Autodesk Fusion 360 part; units mm, degrees
(part 8 of 8)
  line L2633 (-418.8503, 9.35) -> (-418.8503, 6.35)
  line L2634 (-418.8503, 6.35) -> (-415.8503, 6.35)
  line L2635 (-415.8503, 6.35) -> (-415.8503, 9.35)
  line L2636 (-415.8503, 9.35) -> (-412.8503, 9.35)
  line L2637 (-412.8503, 9.35) -> (-412.8503, 6.35)
  line L2638 (-412.8503, 6.35) -> (-409.8503, 6.35)
  line L2639 (-409.8503, 6.35) -> (-409.8503, 9.35)
  line L2640 (-409.8503, 9.35) -> (-406.8503, 9.35)
  line L2641 (-406.8503, 9.35) -> (-406.8503, 6.35)
  line L2642 (-406.8503, 6.35) -> (-403.8503, 6.35)
  line L2643 (-403.8503, 6.35) -> (-403.8503, 9.35)
  line L2644 (-403.8503, 9.35) -> (-400.8503, 9.35)
  line L2645 (-400.8503, 9.35) -> (-400.8503, 6.35)
  line L2646 (-400.8503, 6.35) -> (-397.8503, 6.35)
  line L2647 (-397.8503, 6.35) -> (-397.8503, 9.35)
  line L2648 (-397.8503, 9.35) -> (-394.8503, 9.35)
  line L2649 (-394.8503, 9.35) -> (-394.8503, 6.35)
  line L2650 (-394.8503, 6.35) -> (-391.8503, 6.35)
  line L2651 (-391.8503, 6.35) -> (-391.8503, 9.35)
  line L2652 (-391.8503, 9.35) -> (-388.8503, 9.35)
  line L2653 (-388.8503, 9.35) -> (-388.8503, 6.35)
  line L2654 (-388.8503, 6.35) -> (-385.8503, 6.35)
  line L2655 (-385.8503, 6.35) -> (-385.8503, 9.35)
  line L2656 (-385.8503, 9.35) -> (-382.8503, 9.35)
  line L2657 (-382.8503, 9.35) -> (-382.8503, 6.35)
  line L2658 (-382.8503, 6.35) -> (-379.8503, 6.35)
  line L2659 (-379.8503, 6.35) -> (-379.8503, 9.35)
  line L2660 (-379.8503, 9.35) -> (-376.8503, 9.35)
  line L2661 (-376.8503, 9.35) -> (-376.8503, 6.35)
  line L2662 (-376.8503, 6.35) -> (-373.8503, 6.35)
  line L2663 (-373.8503, 6.35) -> (-373.8503, 9.35)
  line L2664 (-373.8503, 9.35) -> (-370.8503, 9.35)
  line L2665 (-370.8503, 9.35) -> (-370.8503, 6.35)
  line L2666 (-370.8503, 6.35) -> (-367.8503, 6.35)
  line L2667 (-367.8503, 6.35) -> (-367.8503, 9.35)
  line L2668 (-367.8503, 9.35) -> (-364.8503, 9.35)
  line L2669 (-364.8503, 9.35) -> (-364.8503, 6.35)
  line L2670 (-364.8503, 6.35) -> (-361.8503, 6.35)
  line L2671 (-361.8503, 6.35) -> (-361.8503, 9.35)
  line L2672 (-361.8503, 9.35) -> (-358.8503, 9.35)
  line L2673 (-358.8503, 9.35) -> (-358.8503, 6.35)
  line L2674 (-358.8503, 6.35) -> (-355.8503, 6.35)
  line L2675 (-355.8503, 6.35) -> (-355.8503, 9.35)
  line L2676 (-355.8503, 9.35) -> (-352.8503, 9.35)
  line L2677 (-352.8503, 9.35) -> (-352.8503, 6.35)
  line L2678 (-352.8503, 6.35) -> (-349.8503, 6.35)
  line L2679 (-349.8503, 6.35) -> (-349.8503, 9.35)
  line L2680 (-349.8503, 9.35) -> (-346.8503, 9.35)
  line L2681 (-346.8503, 9.35) -> (-346.8503, 6.35)
  line L2682 (-346.8503, 6.35) -> (-343.8503, 6.35)
  line L2683 (-343.8503, 6.35) -> (-343.8503, 9.35)
  line L2684 (-343.8503, 9.35) -> (-340.8503, 9.35)
  line L2685 (-340.8503, 9.35) -> (-340.8503, 6.35)
  line L2686 (-340.8503, 6.35) -> (-337.8503, 6.35)
  line L2687 (-337.8503, 6.35) -> (-337.8503, 9.35)
  line L2688 (-337.8503, 9.35) -> (-334.8503, 9.35)
  line L2689 (-334.8503, 9.35) -> (-334.8503, 6.35)
  line L2690 (-334.8503, 6.35) -> (-331.8503, 6.35)
  line L2691 (-331.8503, 6.35) -> (-331.8503, 9.35)
  line L2692 (-331.8503, 9.35) -> (-327.1003, 9.35)
  line L2693 (-327.1003, 9.35) -> (-327.1003, 6.35)
  line L2694 (-327.1003, 6.35) -> (-322.3503, 6.35)
  line L2695 (-322.3503, 6.35) -> (-322.3503, 10.1)
  line L2696 (-790.6007, 21.35) -> (-790.6007, 24.35)
  line L2697 (-790.6007, 24.35) -> (-791.3507, 24.35)
  line L2698 (-791.3507, 24.35) -> (-791.3507, 20.6)
  line L2699 (-791.3507, 20.6) -> (-794.3507, 20.6)
  line L2700 (-794.3507, 20.6) -> (-794.3507, 16.85)
  line L2701 (-794.3507, 16.85) -> (-791.3507, 16.85)
  line L2702 (-791.3507, 16.85) -> (-791.3507, 13.85)
  line L2703 (-791.3507, 13.85) -> (-794.3507, 13.85)
  line L2704 (-794.3507, 13.85) -> (-794.3507, 10.1)
  line L2705 (-794.3507, 10.1) -> (-791.3507, 10.1)
  line L2706 (-791.3507, 10.1) -> (-791.3507, 6.35)
  line L2707 (-791.3507, 6.35) -> (-790.6007, 6.35)
  line L2708 (-790.6007, 6.35) -> (-790.6007, 9.35)
  line L2709 (-790.6007, 9.35) -> (-786.8506, 9.35)
  line L2710 (-786.8506, 9.35) -> (-786.8506, 6.35)
  line L2711 (-786.8506, 6.35) -> (-783.8506, 6.35)
  line L2712 (-783.8506, 6.35) -> (-783.8506, 9.35)
  line L2713 (-783.8506, 9.35) -> (-780.8506, 9.35)
  line L2714 (-780.8506, 9.35) -> (-780.8506, 6.35)
  line L2715 (-780.8506, 6.35) -> (-777.8506, 6.35)
  line L2716 (-777.8506, 6.35) -> (-777.8506, 9.35)
  line L2717 (-777.8506, 9.35) -> (-774.8506, 9.35)
  line L2718 (-774.8506, 9.35) -> (-774.8506, 6.35)
  line L2719 (-774.8506, 6.35) -> (-771.8506, 6.35)
  line L2720 (-771.8506, 6.35) -> (-771.8506, 9.35)
  line L2721 (-771.8506, 9.35) -> (-768.8506, 9.35)
  line L2722 (-768.8506, 9.35) -> (-768.8506, 6.35)
  line L2723 (-768.8506, 6.35) -> (-765.8506, 6.35)
  line L2724 (-765.8506, 6.35) -> (-765.8506, 9.35)
  line L2725 (-765.8506, 9.35) -> (-762.8506, 9.35)
  line L2726 (-762.8506, 9.35) -> (-762.8506, 6.35)
  line L2727 (-762.8506, 6.35) -> (-759.8506, 6.35)
  line L2728 (-759.8506, 6.35) -> (-759.8506, 9.35)
  line L2729 (-759.8506, 9.35) -> (-756.8506, 9.35)
  line L2730 (-756.8506, 9.35) -> (-756.8506, 6.35)
  line L2731 (-756.8506, 6.35) -> (-753.8506, 6.35)
  line L2732 (-753.8506, 6.35) -> (-753.8506, 9.35)
  line L2733 (-753.8506, 9.35) -> (-750.8506, 9.35)
  line L2734 (-750.8506, 9.35) -> (-750.8506, 6.35)
  line L2735 (-750.8506, 6.35) -> (-747.8506, 6.35)
  line L2736 (-747.8506, 6.35) -> (-747.8506, 9.35)
  line L2737 (-747.8506, 9.35) -> (-744.8506, 9.35)
  line L2738 (-744.8506, 9.35) -> (-744.8506, 6.35)
  line L2739 (-744.8506, 6.35) -> (-741.8506, 6.35)
  line L2740 (-741.8506, 6.35) -> (-741.8506, 9.35)
  line L2741 (-741.8506, 9.35) -> (-738.8506, 9.35)
  line L2742 (-738.8506, 9.35) -> (-738.8506, 6.35)
  line L2743 (-738.8506, 6.35) -> (-735.8506, 6.35)
  line L2744 (-735.8506, 6.35) -> (-735.8506, 9.35)
  line L2745 (-735.8506, 9.35) -> (-732.8506, 9.35)
  line L2746 (-732.8506, 9.35) -> (-732.8506, 6.35)
  line L2747 (-732.8506, 6.35) -> (-729.8506, 6.35)
  line L2748 (-729.8506, 6.35) -> (-729.8506, 9.35)
  line L2749 (-729.8506, 9.35) -> (-726.8506, 9.35)
  line L2750 (-726.8506, 9.35) -> (-726.8506, 6.35)
  line L2751 (-726.8506, 6.35) -> (-723.8506, 6.35)
  line L2752 (-723.8506, 6.35) -> (-723.8506, 9.35)
  line L2753 (-723.8506, 9.35) -> (-720.8506, 9.35)
  line L2754 (-720.8506, 9.35) -> (-720.8506, 6.35)
  line L2755 (-720.8506, 6.35) -> (-717.8506, 6.35)
  line L2756 (-717.8506, 6.35) -> (-717.8506, 9.35)
  line L2757 (-717.8506, 9.35) -> (-714.8506, 9.35)
  line L2758 (-714.8506, 9.35) -> (-714.8506, 6.35)
  line L2759 (-714.8506, 6.35) -> (-711.8506, 6.35)
  line L2760 (-711.8506, 6.35) -> (-711.8506, 9.35)
  line L2761 (-711.8506, 9.35) -> (-708.8506, 9.35)
  line L2762 (-708.8506, 9.35) -> (-708.8506, 6.35)
  line L2763 (-708.8506, 6.35) -> (-705.8506, 6.35)
  line L2764 (-705.8506, 6.35) -> (-705.8506, 9.35)
  line L2765 (-705.8506, 9.35) -> (-702.8506, 9.35)
  line L2766 (-702.8506, 9.35) -> (-702.8506, 6.35)
  line L2767 (-702.8506, 6.35) -> (-699.8506, 6.35)
  line L2768 (-699.8506, 6.35) -> (-699.8506, 9.35)
  line L2769 (-699.8506, 9.35) -> (-696.8506, 9.35)
  line L2770 (-696.8506, 9.35) -> (-696.8506, 6.35)
  line L2771 (-696.8506, 6.35) -> (-693.8506, 6.35)
  line L2772 (-693.8506, 6.35) -> (-693.8506, 9.35)
  line L2773 (-693.8506, 9.35) -> (-690.8506, 9.35)
  line L2774 (-690.8506, 9.35) -> (-690.8506, 6.35)
  line L2775 (-690.8506, 6.35) -> (-687.8506, 6.35)
  line L2776 (-687.8506, 6.35) -> (-687.8506, 9.35)
  line L2777 (-687.8506, 9.35) -> (-684.8506, 9.35)
  line L2778 (-684.8506, 9.35) -> (-684.8506, 6.35)
  line L2779 (-684.8506, 6.35) -> (-681.8506, 6.35)
  line L2780 (-681.8506, 6.35) -> (-681.8506, 9.35)
  line L2781 (-681.8506, 9.35) -> (-678.8506, 9.35)
  line L2782 (-678.8506, 9.35) -> (-678.8506, 6.35)
  line L2783 (-678.8506, 6.35) -> (-675.8506, 6.35)
  line L2784 (-675.8506, 6.35) -> (-675.8506, 9.35)
  line L2785 (-675.8506, 9.35) -> (-672.8506, 9.35)
  line L2786 (-672.8506, 9.35) -> (-672.8506, 6.35)
  line L2787 (-672.8506, 6.35) -> (-669.8506, 6.35)
  line L2788 (-669.8506, 6.35) -> (-669.8506, 9.35)
  line L2789 (-669.8506, 9.35) -> (-666.8505, 9.35)
  line L2790 (-666.8505, 9.35) -> (-666.8505, 6.35)
  line L2791 (-666.8505, 6.35) -> (-663.8505, 6.35)
  line L2792 (-663.8505, 6.35) -> (-663.8505, 9.35)
  line L2793 (-663.8505, 9.35) -> (-660.8505, 9.35)
  line L2794 (-660.8505, 9.35) -> (-660.8505, 6.35)
  line L2795 (-660.8505, 6.35) -> (-657.8505, 6.35)
  line L2796 (-657.8505, 6.35) -> (-657.8505, 9.35)
  line L2797 (-657.8505, 9.35) -> (-654.8505, 9.35)
  line L2798 (-654.8505, 9.35) -> (-654.8505, 6.35)
  line L2799 (-654.8505, 6.35) -> (-651.8505, 6.35)
  line L2800 (-651.8505, 6.35) -> (-651.8505, 9.35)
  line L2801 (-651.8505, 9.35) -> (-648.8505, 9.35)
  line L2802 (-648.8505, 9.35) -> (-648.8505, 6.35)
  line L2803 (-648.8505, 6.35) -> (-645.8505, 6.35)
  line L2804 (-645.8505, 6.35) -> (-645.8505, 9.35)
  line L2805 (-645.8505, 9.35) -> (-642.1005, 9.35)
  line L2806 (-642.1005, 9.35) -> (-642.1005, 6.35)
  line L2807 (-642.1005, 6.35) -> (-641.3505, 6.35)
  line L2808 (-641.3505, 6.35) -> (-641.3505, 10.1)
  line L2809 (-641.3505, 10.1) -> (-638.3505, 10.1)
  line L2810 (-638.3505, 10.1) -> (-638.3505, 13.85)
  line L2811 (-638.3505, 13.85) -> (-641.3505, 13.85)
  line L2812 (-641.3505, 13.85) -> (-641.3505, 16.85)
  line L2813 (-641.3505, 16.85) -> (-638.3505, 16.85)
  line L2814 (-638.3505, 16.85) -> (-638.3505, 20.6)
  line L2815 (-638.3505, 20.6) -> (-641.3505, 20.6)
  line L2816 (-641.3505, 20.6) -> (-641.3505, 24.35)
  line L2817 (-641.3505, 24.35) -> (-642.1005, 24.35)
  line L2818 (-642.1005, 24.35) -> (-642.1005, 21.35)
  line L2819 (-642.1005, 21.35) -> (-645.8505, 21.35)
  line L2820 (-645.8505, 21.35) -> (-645.8505, 24.35)
  line L2821 (-645.8505, 24.35) -> (-648.8505, 24.35)
  line L2822 (-648.8505, 24.35) -> (-648.8505, 21.35)
  line L2823 (-648.8505, 21.35) -> (-651.8505, 21.35)
  line L2824 (-651.8505, 21.35) -> (-651.8505, 24.35)
  line L2825 (-651.8505, 24.35) -> (-654.8505, 24.35)
  line L2826 (-654.8505, 24.35) -> (-654.8505, 21.35)
  line L2827 (-654.8505, 21.35) -> (-657.8505, 21.35)
  line L2828 (-657.8505, 21.35) -> (-657.8505, 24.35)
  line L2829 (-657.8505, 24.35) -> (-660.8505, 24.35)
  line L2830 (-660.8505, 24.35) -> (-660.8505, 21.35)
  line L2831 (-660.8505, 21.35) -> (-663.8505, 21.35)
  line L2832 (-663.8505, 21.35) -> (-663.8505, 24.35)
  line L2833 (-663.8505, 24.35) -> (-666.8505, 24.35)
  line L2834 (-666.8505, 24.35) -> (-666.8505, 21.35)
  line L2835 (-666.8505, 21.35) -> (-669.8506, 21.35)
  line L2836 (-669.8506, 21.35) -> (-669.8506, 24.35)
  line L2837 (-669.8506, 24.35) -> (-672.8506, 24.35)
  line L2838 (-672.8506, 24.35) -> (-672.8506, 21.35)
  line L2839 (-672.8506, 21.35) -> (-675.8506, 21.35)
  line L2840 (-675.8506, 21.35) -> (-675.8506, 24.35)
  line L2841 (-675.8506, 24.35) -> (-678.8506, 24.35)
  line L2842 (-678.8506, 24.35) -> (-678.8506, 21.35)
  line L2843 (-678.8506, 21.35) -> (-681.8506, 21.35)
  line L2844 (-681.8506, 21.35) -> (-681.8506, 24.35)
  line L2845 (-681.8506, 24.35) -> (-684.8506, 24.35)
  line L2846 (-684.8506, 24.35) -> (-684.8506, 21.35)
  line L2847 (-684.8506, 21.35) -> (-687.8506, 21.35)
  line L2848 (-687.8506, 21.35) -> (-687.8506, 24.35)
  line L2849 (-687.8506, 24.35) -> (-690.8506, 24.35)
  line L2850 (-690.8506, 24.35) -> (-690.8506, 21.35)
  line L2851 (-690.8506, 21.35) -> (-693.8506, 21.35)
  line L2852 (-693.8506, 21.35) -> (-693.8506, 24.35)
  line L2853 (-693.8506, 24.35) -> (-696.8506, 24.35)
  line L2854 (-696.8506, 24.35) -> (-696.8506, 21.35)
  line L2855 (-696.8506, 21.35) -> (-699.8506, 21.35)
  line L2856 (-699.8506, 21.35) -> (-699.8506, 24.35)
  line L2857 (-699.8506, 24.35) -> (-702.8506, 24.35)
  line L2858 (-702.8506, 24.35) -> (-702.8506, 21.35)
  line L2859 (-702.8506, 21.35) -> (-705.8506, 21.35)
  line L2860 (-705.8506, 21.35) -> (-705.8506, 24.35)
  line L2861 (-705.8506, 24.35) -> (-708.8506, 24.35)
  line L2862 (-708.8506, 24.35) -> (-708.8506, 21.35)
  line L2863 (-708.8506, 21.35) -> (-711.8506, 21.35)
  line L2864 (-711.8506, 21.35) -> (-711.8506, 24.35)
  line L2865 (-711.8506, 24.35) -> (-714.8506, 24.35)
  line L2866 (-714.8506, 24.35) -> (-714.8506, 21.35)
  line L2867 (-714.8506, 21.35) -> (-717.8506, 21.35)
  line L2868 (-717.8506, 21.35) -> (-717.8506, 24.35)
  line L2869 (-717.8506, 24.35) -> (-720.8506, 24.35)
  line L2870 (-720.8506, 24.35) -> (-720.8506, 21.35)
  line L2871 (-720.8506, 21.35) -> (-723.8506, 21.35)
  line L2872 (-723.8506, 21.35) -> (-723.8506, 24.35)
  line L2873 (-723.8506, 24.35) -> (-726.8506, 24.35)
  line L2874 (-726.8506, 24.35) -> (-726.8506, 21.35)
  line L2875 (-726.8506, 21.35) -> (-729.8506, 21.35)
  line L2876 (-729.8506, 21.35) -> (-729.8506, 24.35)
  line L2877 (-729.8506, 24.35) -> (-732.8506, 24.35)
  line L2878 (-732.8506, 24.35) -> (-732.8506, 21.35)
  line L2879 (-732.8506, 21.35) -> (-735.8506, 21.35)
  line L2880 (-735.8506, 21.35) -> (-735.8506, 24.35)
  line L2881 (-735.8506, 24.35) -> (-738.8506, 24.35)
  line L2882 (-738.8506, 24.35) -> (-738.8506, 21.35)
  line L2883 (-738.8506, 21.35) -> (-741.8506, 21.35)
  line L2884 (-741.8506, 21.35) -> (-741.8506, 24.35)
  line L2885 (-741.8506, 24.35) -> (-744.8506, 24.35)
  line L2886 (-744.8506, 24.35) -> (-744.8506, 21.35)
  line L2887 (-744.8506, 21.35) -> (-747.8506, 21.35)
  line L2888 (-747.8506, 21.35) -> (-747.8506, 24.35)
  line L2889 (-747.8506, 24.35) -> (-750.8506, 24.35)
  line L2890 (-750.8506, 24.35) -> (-750.8506, 21.35)
  line L2891 (-750.8506, 21.35) -> (-753.8506, 21.35)
  line L2892 (-753.8506, 21.35) -> (-753.8506, 24.35)
  line L2893 (-753.8506, 24.35) -> (-756.8506, 24.35)
  line L2894 (-756.8506, 24.35) -> (-756.8506, 21.35)
  line L2895 (-756.8506, 21.35) -> (-759.8506, 21.35)
  line L2896 (-759.8506, 21.35) -> (-759.8506, 24.35)
  line L2897 (-759.8506, 24.35) -> (-762.8506, 24.35)
  line L2898 (-762.8506, 24.35) -> (-762.8506, 21.35)
  line L2899 (-762.8506, 21.35) -> (-765.8506, 21.35)
  line L2900 (-765.8506, 21.35) -> (-765.8506, 24.35)
  line L2901 (-765.8506, 24.35) -> (-768.8506, 24.35)
  line L2902 (-768.8506, 24.35) -> (-768.8506, 21.35)
  line L2903 (-768.8506, 21.35) -> (-771.8506, 21.35)
  line L2904 (-771.8506, 21.35) -> (-771.8506, 24.35)
  line L2905 (-771.8506, 24.35) -> (-774.8506, 24.35)
  line L2906 (-774.8506, 24.35) -> (-774.8506, 21.35)
  line L2907 (-774.8506, 21.35) -> (-777.8506, 21.35)
  line L2908 (-777.8506, 21.35) -> (-777.8506, 24.35)
  line L2909 (-777.8506, 24.35) -> (-780.8506, 24.35)
  line L2910 (-780.8506, 24.35) -> (-780.8506, 21.35)
  line L2911 (-780.8506, 21.35) -> (-783.8506, 21.35)
  line L2912 (-783.8506, 21.35) -> (-783.8506, 24.35)
  line L2913 (-783.8506, 24.35) -> (-786.8506, 24.35)
  line L2914 (-786.8506, 24.35) -> (-786.8506, 21.35)
  line L2915 (-786.8506, 21.35) -> (-790.6007, 21.35)
  line L2916 (-727.1005, 38.1605) -> (-712.1005, 38.1605)
  line L2917 (-712.1005, 38.1605) -> (-712.1005, 29.1605)
  line L2918 (-712.1005, 29.1605) -> (-727.1005, 29.1605)
  line L2919 (-727.1005, 29.1605) -> (-727.1005, 38.1605)
  line L2920 (-641.3505, 34.85) -> (-638.3505, 34.85)
  line L2921 (-638.3505, 34.85) -> (-638.3505, 38.6)
  line L2922 (-638.3505, 38.6) -> (-641.3505, 38.6)
  line L2923 (-641.3505, 38.6) -> (-641.3505, 42.35)
  line L2924 (-641.3505, 42.35) -> (-642.1005, 42.35)
  line L2925 (-642.1005, 42.35) -> (-642.1005, 39.35)
  line L2926 (-642.1005, 39.35) -> (-645.8505, 39.35)
  line L2927 (-645.8505, 39.35) -> (-645.8505, 42.35)
  line L2928 (-645.8505, 42.35) -> (-648.8505, 42.35)
  line L2929 (-648.8505, 42.35) -> (-648.8505, 39.35)
  line L2930 (-648.8505, 39.35) -> (-651.8505, 39.35)
  line L2931 (-651.8505, 39.35) -> (-651.8505, 42.35)
  line L2932 (-651.8505, 42.35) -> (-654.8505, 42.35)
  line L2933 (-654.8505, 42.35) -> (-654.8505, 39.35)
  line L2934 (-654.8505, 39.35) -> (-657.8505, 39.35)
  line L2935 (-657.8505, 39.35) -> (-657.8505, 42.35)
  line L2936 (-657.8505, 42.35) -> (-660.8505, 42.35)
  line L2937 (-660.8505, 42.35) -> (-660.8505, 39.35)
  line L2938 (-660.8505, 39.35) -> (-663.8505, 39.35)
  line L2939 (-663.8505, 39.35) -> (-663.8505, 42.35)
  line L2940 (-663.8505, 42.35) -> (-666.8505, 42.35)
  line L2941 (-666.8505, 42.35) -> (-666.8505, 39.35)
  line L2942 (-666.8505, 39.35) -> (-669.8506, 39.35)
  line L2943 (-669.8506, 39.35) -> (-669.8506, 42.35)
  line L2944 (-669.8506, 42.35) -> (-672.8506, 42.35)
  line L2945 (-672.8506, 42.35) -> (-672.8506, 39.35)
  line L2946 (-672.8506, 39.35) -> (-675.8506, 39.35)
  line L2947 (-675.8506, 39.35) -> (-675.8506, 42.35)
  line L2948 (-675.8506, 42.35) -> (-678.8506, 42.35)
  line L2949 (-678.8506, 42.35) -> (-678.8506, 39.35)
  line L2950 (-678.8506, 39.35) -> (-681.8506, 39.35)
  line L2951 (-681.8506, 39.35) -> (-681.8506, 42.35)
  line L2952 (-681.8506, 42.35) -> (-684.8506, 42.35)
  line L2953 (-684.8506, 42.35) -> (-684.8506, 39.35)
  line L2954 (-684.8506, 39.35) -> (-687.8506, 39.35)
  line L2955 (-687.8506, 39.35) -> (-687.8506, 42.35)
  line L2956 (-687.8506, 42.35) -> (-690.8506, 42.35)
  line L2957 (-690.8506, 42.35) -> (-690.8506, 39.35)
  line L2958 (-690.8506, 39.35) -> (-693.8506, 39.35)
  line L2959 (-693.8506, 39.35) -> (-693.8506, 42.35)
  line L2960 (-693.8506, 42.35) -> (-696.8506, 42.35)
  line L2961 (-696.8506, 42.35) -> (-696.8506, 39.35)
  line L2962 (-696.8506, 39.35) -> (-699.8506, 39.35)
  line L2963 (-699.8506, 39.35) -> (-699.8506, 42.35)
  line L2964 (-699.8506, 42.35) -> (-702.8506, 42.35)
  line L2965 (-702.8506, 42.35) -> (-702.8506, 39.35)
  line L2966 (-702.8506, 39.35) -> (-705.8506, 39.35)
  line L2967 (-705.8506, 39.35) -> (-705.8506, 42.35)
  line L2968 (-705.8506, 42.35) -> (-708.8506, 42.35)
  line L2969 (-708.8506, 42.35) -> (-708.8506, 39.35)
  line L2970 (-708.8506, 39.35) -> (-711.8506, 39.35)
  line L2971 (-711.8506, 39.35) -> (-711.8506, 42.35)
  line L2972 (-711.8506, 42.35) -> (-714.8506, 42.35)
  line L2973 (-714.8506, 42.35) -> (-714.8506, 39.35)
  line L2974 (-714.8506, 39.35) -> (-717.8506, 39.35)
  line L2975 (-717.8506, 39.35) -> (-717.8506, 42.35)
  line L2976 (-717.8506, 42.35) -> (-720.8506, 42.35)
  line L2977 (-720.8506, 42.35) -> (-720.8506, 39.35)
  line L2978 (-720.8506, 39.35) -> (-723.8506, 39.35)
  line L2979 (-723.8506, 39.35) -> (-723.8506, 42.35)
  line L2980 (-723.8506, 42.35) -> (-726.8506, 42.35)
  line L2981 (-726.8506, 42.35) -> (-726.8506, 39.35)
  line L2982 (-726.8506, 39.35) -> (-729.8506, 39.35)
  line L2983 (-729.8506, 39.35) -> (-729.8506, 42.35)
  line L2984 (-729.8506, 42.35) -> (-732.8506, 42.35)
  line L2985 (-732.8506, 42.35) -> (-732.8506, 39.35)
  line L2986 (-732.8506, 39.35) -> (-735.8506, 39.35)
  line L2987 (-735.8506, 39.35) -> (-735.8506, 42.35)
  line L2988 (-735.8506, 42.35) -> (-738.8506, 42.35)
  line L2989 (-738.8506, 42.35) -> (-738.8506, 39.35)
  line L2990 (-738.8506, 39.35) -> (-741.8506, 39.35)
  line L2991 (-741.8506, 39.35) -> (-741.8506, 42.35)
  line L2992 (-741.8506, 42.35) -> (-744.8506, 42.35)
  line L2993 (-744.8506, 42.35) -> (-744.8506, 39.35)
  line L2994 (-744.8506, 39.35) -> (-747.8506, 39.35)
  line L2995 (-747.8506, 39.35) -> (-747.8506, 42.35)
  line L2996 (-747.8506, 42.35) -> (-750.8506, 42.35)
  line L2997 (-750.8506, 42.35) -> (-750.8506, 39.35)
  line L2998 (-750.8506, 39.35) -> (-753.8506, 39.35)
  line L2999 (-753.8506, 39.35) -> (-753.8506, 42.35)
  line L3000 (-753.8506, 42.35) -> (-756.8506, 42.35)
  line L3001 (-756.8506, 42.35) -> (-756.8506, 39.35)
  line L3002 (-756.8506, 39.35) -> (-759.8506, 39.35)
  line L3003 (-759.8506, 39.35) -> (-759.8506, 42.35)
  line L3004 (-759.8506, 42.35) -> (-762.8506, 42.35)
  line L3005 (-762.8506, 42.35) -> (-762.8506, 39.35)
  line L3006 (-762.8506, 39.35) -> (-765.8506, 39.35)
  line L3007 (-765.8506, 39.35) -> (-765.8506, 42.35)
  line L3008 (-765.8506, 42.35) -> (-768.8506, 42.35)
  line L3009 (-768.8506, 42.35) -> (-768.8506, 39.35)
  line L3010 (-768.8506, 39.35) -> (-771.8506, 39.35)
  line L3011 (-771.8506, 39.35) -> (-771.8506, 42.35)
  line L3012 (-771.8506, 42.35) -> (-774.8506, 42.35)
  line L3013 (-774.8506, 42.35) -> (-774.8506, 39.35)
  line L3014 (-774.8506, 39.35) -> (-777.8506, 39.35)
  line L3015 (-777.8506, 39.35) -> (-777.8506, 42.35)
  line L3016 (-777.8506, 42.35) -> (-780.8506, 42.35)
  line L3017 (-780.8506, 42.35) -> (-780.8506, 39.35)
  line L3018 (-780.8506, 39.35) -> (-783.8506, 39.35)
  line L3019 (-783.8506, 39.35) -> (-783.8506, 42.35)
  line L3020 (-783.8506, 42.35) -> (-786.8506, 42.35)
  line L3021 (-786.8506, 42.35) -> (-786.8506, 39.35)
  line L3022 (-786.8506, 39.35) -> (-790.6007, 39.35)
  line L3023 (-790.6007, 39.35) -> (-790.6007, 42.35)
  line L3024 (-790.6007, 42.35) -> (-791.3507, 42.35)
  line L3025 (-791.3507, 42.35) -> (-791.3507, 38.6)
  line L3026 (-791.3507, 38.6) -> (-794.3507, 38.6)
  line L3027 (-794.3507, 38.6) -> (-794.3507, 34.85)
  line L3028 (-794.3507, 34.85) -> (-791.3507, 34.85)
  line L3029 (-791.3507, 34.85) -> (-791.3507, 31.85)
  line L3030 (-791.3507, 31.85) -> (-794.3507, 31.85)
  line L3031 (-794.3507, 31.85) -> (-794.3507, 28.1)
  line L3032 (-794.3507, 28.1) -> (-791.3507, 28.1)
  line L3033 (-791.3507, 28.1) -> (-791.3507, 24.35)
  line L3034 (-791.3507, 24.35) -> (-790.6007, 24.35)
  line L3035 (-790.6007, 24.35) -> (-790.6007, 27.35)
  line L3036 (-790.6007, 27.35) -> (-786.8506, 27.35)
  line L3037 (-786.8506, 27.35) -> (-786.8506, 24.35)
  line L3038 (-786.8506, 24.35) -> (-783.8506, 24.35)
  line L3039 (-783.8506, 24.35) -> (-783.8506, 27.35)
  line L3040 (-783.8506, 27.35) -> (-780.8506, 27.35)
  line L3041 (-780.8506, 27.35) -> (-780.8506, 24.35)
  line L3042 (-780.8506, 24.35) -> (-777.8506, 24.35)
  line L3043 (-777.8506, 24.35) -> (-777.8506, 27.35)
  line L3044 (-777.8506, 27.35) -> (-774.8506, 27.35)
  line L3045 (-774.8506, 27.35) -> (-774.8506, 24.35)
  line L3046 (-774.8506, 24.35) -> (-771.8506, 24.35)
  line L3047 (-771.8506, 24.35) -> (-771.8506, 27.35)
  line L3048 (-771.8506, 27.35) -> (-768.8506, 27.35)
  line L3049 (-768.8506, 27.35) -> (-768.8506, 24.35)
  line L3050 (-768.8506, 24.35) -> (-765.8506, 24.35)
  line L3051 (-765.8506, 24.35) -> (-765.8506, 27.35)
  line L3052 (-765.8506, 27.35) -> (-762.8506, 27.35)
  line L3053 (-762.8506, 27.35) -> (-762.8506, 24.35)
  line L3054 (-762.8506, 24.35) -> (-759.8506, 24.35)
  line L3055 (-759.8506, 24.35) -> (-759.8506, 27.35)
  line L3056 (-759.8506, 27.35) -> (-756.8506, 27.35)
  line L3057 (-756.8506, 27.35) -> (-756.8506, 24.35)
  line L3058 (-756.8506, 24.35) -> (-753.8506, 24.35)
  line L3059 (-753.8506, 24.35) -> (-753.8506, 27.35)
  line L3060 (-753.8506, 27.35) -> (-750.8506, 27.35)
  line L3061 (-750.8506, 27.35) -> (-750.8506, 24.35)
  line L3062 (-750.8506, 24.35) -> (-747.8506, 24.35)
  line L3063 (-747.8506, 24.35) -> (-747.8506, 27.35)
  line L3064 (-747.8506, 27.35) -> (-744.8506, 27.35)
  line L3065 (-744.8506, 27.35) -> (-744.8506, 24.35)
  line L3066 (-744.8506, 24.35) -> (-741.8506, 24.35)
  line L3067 (-741.8506, 24.35) -> (-741.8506, 27.35)
  line L3068 (-741.8506, 27.35) -> (-738.8506, 27.35)
  line L3069 (-738.8506, 27.35) -> (-738.8506, 24.35)
  line L3070 (-738.8506, 24.35) -> (-735.8506, 24.35)
  line L3071 (-735.8506, 24.35) -> (-735.8506, 27.35)
  line L3072 (-735.8506, 27.35) -> (-732.8506, 27.35)
  line L3073 (-732.8506, 27.35) -> (-732.8506, 24.35)
  line L3074 (-732.8506, 24.35) -> (-729.8506, 24.35)
  line L3075 (-729.8506, 24.35) -> (-729.8506, 27.35)
  line L3076 (-729.8506, 27.35) -> (-726.8506, 27.35)
  line L3077 (-726.8506, 27.35) -> (-726.8506, 24.35)
  line L3078 (-726.8506, 24.35) -> (-723.8506, 24.35)
  line L3079 (-723.8506, 24.35) -> (-723.8506, 27.35)
  line L3080 (-723.8506, 27.35) -> (-720.8506, 27.35)
  line L3081 (-720.8506, 27.35) -> (-720.8506, 24.35)
  line L3082 (-720.8506, 24.35) -> (-717.8506, 24.35)
  line L3083 (-717.8506, 24.35) -> (-717.8506, 27.35)
  line L3084 (-717.8506, 27.35) -> (-714.8506, 27.35)
  line L3085 (-714.8506, 27.35) -> (-714.8506, 24.35)
  line L3086 (-714.8506, 24.35) -> (-711.8506, 24.35)
  line L3087 (-711.8506, 24.35) -> (-711.8506, 27.35)
  line L3088 (-711.8506, 27.35) -> (-708.8506, 27.35)
  line L3089 (-708.8506, 27.35) -> (-708.8506, 24.35)
  line L3090 (-708.8506, 24.35) -> (-705.8506, 24.35)
  line L3091 (-705.8506, 24.35) -> (-705.8506, 27.35)
  line L3092 (-705.8506, 27.35) -> (-702.8506, 27.35)
  line L3093 (-702.8506, 27.35) -> (-702.8506, 24.35)
  line L3094 (-702.8506, 24.35) -> (-699.8506, 24.35)
  line L3095 (-699.8506, 24.35) -> (-699.8506, 27.35)
  line L3096 (-699.8506, 27.35) -> (-696.8506, 27.35)
  line L3097 (-696.8506, 27.35) -> (-696.8506, 24.35)
  line L3098 (-696.8506, 24.35) -> (-693.8506, 24.35)
  line L3099 (-693.8506, 24.35) -> (-693.8506, 27.35)
  line L3100 (-693.8506, 27.35) -> (-690.8506, 27.35)
  line L3101 (-690.8506, 27.35) -> (-690.8506, 24.35)
  line L3102 (-690.8506, 24.35) -> (-687.8506, 24.35)
  line L3103 (-687.8506, 24.35) -> (-687.8506, 27.35)
  line L3104 (-687.8506, 27.35) -> (-684.8506, 27.35)
  line L3105 (-684.8506, 27.35) -> (-684.8506, 24.35)
  line L3106 (-684.8506, 24.35) -> (-681.8506, 24.35)
  line L3107 (-681.8506, 24.35) -> (-681.8506, 27.35)
  line L3108 (-681.8506, 27.35) -> (-678.8506, 27.35)
  line L3109 (-678.8506, 27.35) -> (-678.8506, 24.35)
  line L3110 (-678.8506, 24.35) -> (-675.8506, 24.35)
  line L3111 (-675.8506, 24.35) -> (-675.8506, 27.35)
  line L3112 (-675.8506, 27.35) -> (-672.8506, 27.35)
  line L3113 (-672.8506, 27.35) -> (-672.8506, 24.35)
  line L3114 (-672.8506, 24.35) -> (-669.8506, 24.35)
  line L3115 (-669.8506, 24.35) -> (-669.8506, 27.35)
  line L3116 (-669.8506, 27.35) -> (-666.8505, 27.35)
  line L3117 (-666.8505, 27.35) -> (-666.8505, 24.35)
  line L3118 (-666.8505, 24.35) -> (-663.8505, 24.35)
  line L3119 (-663.8505, 24.35) -> (-663.8505, 27.35)
  line L3120 (-663.8505, 27.35) -> (-660.8505, 27.35)
  line L3121 (-660.8505, 27.35) -> (-660.8505, 24.35)
  line L3122 (-660.8505, 24.35) -> (-657.8505, 24.35)
  line L3123 (-657.8505, 24.35) -> (-657.8505, 27.35)
  line L3124 (-657.8505, 27.35) -> (-654.8505, 27.35)
  line L3125 (-654.8505, 27.35) -> (-654.8505, 24.35)
  line L3126 (-654.8505, 24.35) -> (-651.8505, 24.35)
  line L3127 (-651.8505, 24.35) -> (-651.8505, 27.35)
  line L3128 (-651.8505, 27.35) -> (-648.8505, 27.35)
  line L3129 (-648.8505, 27.35) -> (-648.8505, 24.35)
  line L3130 (-648.8505, 24.35) -> (-645.8505, 24.35)
  line L3131 (-645.8505, 24.35) -> (-645.8505, 27.35)
  line L3132 (-645.8505, 27.35) -> (-642.1005, 27.35)
  line L3133 (-642.1005, 27.35) -> (-642.1005, 24.35)
  line L3134 (-642.1005, 24.35) -> (-641.3505, 24.35)
  line L3135 (-641.3505, 24.35) -> (-641.3505, 28.1)
  line L3136 (-641.3505, 28.1) -> (-638.3505, 28.1)
  line L3137 (-638.3505, 28.1) -> (-638.3505, 31.85)
  line L3138 (-638.3505, 31.85) -> (-641.3505, 31.85)
  line L3139 (-641.3505, 31.85) -> (-641.3505, 34.85)
  circle A0 centre (-110.4882, 52.6046) radius 2.5
  circle A1 centre (-197.9882, 140.1046) radius 2.5
  circle A2 centre (-210.4882, 152.6046) radius 2.5
  circle A3 centre (-122.9882, 65.1046) radius 2.5
  circle A4 centre (-122.9882, 140.1046) radius 2.5
  circle A5 centre (-197.9882, 65.1046) radius 2.5
  circle A6 centre (-210.4882, 52.6046) radius 2.5
  circle A7 centre (-110.4882, 152.6046) radius 2.5
  circle A8 through (-107.9882, 52.6046, -3) (-111.7382, 54.7696, -3) (-111.7382, 50.4395, -3)
  circle A9 through (-195.4882, 140.1046, -3) (-199.2382, 142.2696, -3) (-199.2382, 137.9395, -3)
  circle A10 through (-207.9882, 152.6046, -3) (-211.7382, 154.7696, -3) (-211.7382, 150.4395, -3)
  circle A11 through (-120.4882, 65.1046, -3) (-124.2382, 67.2696, -3) (-124.2382, 62.9395, -3)
  circle A12 through (-120.4882, 140.1046, -3) (-124.2382, 142.2696, -3) (-124.2382, 137.9395, -3)
  circle A13 through (-195.4882, 65.1046, -3) (-199.2382, 67.2696, -3) (-199.2382, 62.9395, -3)
  circle A14 through (-207.9882, 52.6046, -3) (-211.7382, 54.7696, -3) (-211.7382, 50.4395, -3)
  circle A15 through (-107.9882, 152.6046, -3) (-111.7382, 154.7696, -3) (-111.7382, 150.4395, -3)
